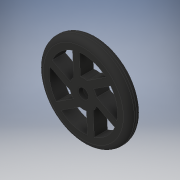
# Autodesk Inventor part: Scooter Wheel
Saved by Autodesk Inventor 2017 (Build 210142000, 142)
## iProperties
Created: 2018-10-18
Part Number: Scooter Wheel
Material: Rubber
Document SubType Name: Modeling
Designer: Administrator
Density: 0.93 g/cm^3
Appearance: Rubber - Black
Author: Administrator
Autodesk Inventor part; units mm, degrees
ref_plane "YZ Plane" through (0, 0, 0) normal (1, 0, 0) x (0, 1, 0)
ref_plane "XZ Plane" through (0, 0, 0) normal (0, 1, 0) x (-1, 0, 0)
ref_plane "XY Plane" through (0, 0, 0) normal (0, 0, 1) x (1, 0, 0)
sketch "Sketch1" plane through (0, 0, 0) normal (0, 0, 1) x (1, 0, 0)
  circle A0 centre (0, 0) radius 4
  circle A1 centre (0, 0) radius 100
  dimension "d0" = 8
  dimension "d1" = 200
  constraints: 2 centre point, 2 coincident
  measures "d0" diameter of A0
  measures "d1" diameter of A1
extrude "Extrusion1" add sketch "Sketch1" along normal blind 29
fillet "Fillet1" radius 12 2 edges at (-100, 0, 29) (-100, 0, 0)
sketch "Sketch2" plane through (0, 0, 29) normal (0, 0, 1) x (1, 0, 0)
  circle A0 centre (0, 0) radius 88 projected
  line L0 (9.0297, 17.8456) -> (73.5273, -14.7895)
  line L1 (19.5363, -4.2815) -> (69.0295, -29.3245)
  arc A1 (19.5363, -4.2815) -> (9.0297, 17.8456) centre (0, 0) ccw
  arc A2 (69.0295, -29.3245) -> (73.5273, -14.7895) centre (0, 0) ccw
  line L2 (13.4761, 14.7782) -> (59.9105, 45.119)
  arc A3 (13.4761, 14.7782) -> (-10.9399, 16.7427) centre (0, 0) ccw
  arc A4 (59.9105, 45.119) -> (49.5718, 56.2818) centre (0, 0) ccw
  line L3 (-10.9399, 16.7427) -> (49.5718, 56.2818)
  line L4 (-6.0602, 19.0597) -> (-9.119, 74.4436)
  arc A5 (-6.0602, 19.0597) -> (-19.9696, -1.1029) centre (0, 0) ccw
  arc A6 (-9.119, 74.4436) -> (-23.9556, 71.0713) centre (0, 0) ccw
  line L5 (-19.9696, -1.1029) -> (-23.9556, 71.0713)
  line L6 (-19.5363, 4.2815) -> (-69.0295, 29.3245)
  arc A7 (-19.5363, 4.2815) -> (-9.0297, -17.8456) centre (0, 0) ccw
  arc A8 (-69.0295, 29.3245) -> (-73.5273, 14.7895) centre (0, 0) ccw
  line L7 (-9.0297, -17.8456) -> (-73.5273, 14.7895)
  line L8 (-13.4761, -14.7782) -> (-59.9105, -45.119)
  arc A9 (-13.4761, -14.7782) -> (10.9399, -16.7427) centre (0, 0) ccw
  arc A10 (-59.9105, -45.119) -> (-49.5718, -56.2818) centre (0, 0) ccw
  line L9 (10.9399, -16.7427) -> (-49.5718, -56.2818)
  line L10 (6.0602, -19.0597) -> (9.119, -74.4436)
  arc A11 (6.0602, -19.0597) -> (19.9696, 1.1029) centre (0, 0) ccw
  arc A12 (9.119, -74.4436) -> (23.9556, -71.0713) centre (0, 0) ccw
  line L11 (19.9696, 1.1029) -> (23.9556, -71.0713)
  circle A13 centre (0, 0) radius 4 projected
  circle A14 centre (0, 0) radius 75
  dimension "d7" = 15
  dimension "d8" = 75
  dimension "d9" = 20
  dimension "d12" = 360
  constraints: 24 end point, 24 point on circle, 12 centre point, 8 coincident, 1 parallel, 64 other
  measures "d7" distance between parallel lines of L1 L0
  measures "d8" radius of A2
  measures "d9" radius of A1
extrude "Extrusion2" cut sketch "Sketch2" against normal through all contours A1 A11 A9 A7 A5 A3 | L2 A14 L0 | L4 A14 L3 | A14 L11 L1 | L6 A14 L5 | A14 L9 L10 | L8 A14 L7
sketch "Sketch3" plane through (0, 0, 29) normal (0, 0, 1) x (1, 0, 0)
  circle A0 centre (0, 0) radius 30
  circle A1 centre (0, 0) radius 20 projected
  dimension "d16" = 60
  constraints: 1 centre point, 1 coincident
  measures "d16" diameter of A0
extrude "Extrusion3" add sketch "Sketch3" against normal blind 29
sketch "Sketch4" plane through (0, 0, 29) normal (0, 0, 1) x (1, 0, 0)
  circle A0 centre (0, 0) radius 20 projected
  circle A1 centre (0, 0) radius 4
  dimension "d19" = 8
  constraints: 1 centre point, 1 coincident
  measures "d19" diameter of A1
extrude "Extrusion4" add sketch "Sketch4" against normal blind 29
sketch "Sketch5" plane through (0, 0, 29) normal (0, 0, 1) x (1, 0, 0)
  circle A0 centre (0, 0) radius 4 projected
  circle A1 centre (0, 0) radius 11
  dimension "d22" = 22
  constraints: 1 centre point, 1 coincident
  measures "d22" diameter of A1
extrude "Extrusion5" cut sketch "Sketch5" against normal blind 10
sketch "Sketch7" plane through (0, 0, 0) normal (0, 0, -1) x (-1, 0, 0)
  circle A0 centre (0, 0) radius 4 projected
  circle A1 centre (0, 0) radius 11
  dimension "d25" = 22
  constraints: 1 centre point, 1 coincident
  measures "d25" diameter of A1
extrude "Extrusion6" cut sketch "Sketch7" against normal blind 10
body "Solid1"
